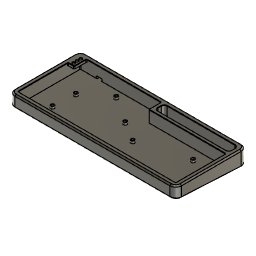
mfrv4n (Autodesk Fusion 360 design; units mm, degrees)
Autodesk Fusion 360 part; units mm, degrees
note: some values were not read from the file. Chosen so that the rebuilt part matches the saved one: a direction. Set by a fixed rule: which sketch regions a step uses.
sketch "PCB Plane Sketch" plane through (0, 0, 0) normal (0, 0, 1) x (1, 0, 0)
  line L0 (0, 0) -> (242.8875, 0) construction
  line L1 (242.8875, 0) -> (242.8875, 76.2) construction
  line L2 (0, 76.2) -> (0, 0) construction
  line L3 (0, 76.2) -> (9.525, 76.2) construction
  line L4 (123.825, 76.2) -> (123.825, 95.25) construction
  line L5 (123.825, 95.25) -> (0, 95.25) construction
  line L6 (0, 95.25) -> (0, 76.2) construction
  line L7 (0, 95.25) -> (9.525, 95.25) construction
  line L8 (9.525, 95.25) -> (9.525, 76.2) construction
  line L9 (9.525, 76.2) -> (0, 76.2) construction
  line L10 (0, 76.2) -> (0, 95.25) construction
  line L11 (242.8875, 76.2) -> (123.825, 76.2) construction
  line L12 (9.525, 76.2) -> (0, 76.2) construction
  line L13 (-0.5, 76.2) -> (-0.5, -0.5)
  line L14 (-0.5, -0.5) -> (243.3875, -0.5)
  line L15 (243.3875, -0.5) -> (243.3875, 76.7)
  line L16 (243.3875, 76.7) -> (124.325, 76.7)
  line L17 (124.325, 76.7) -> (124.325, 95.75)
  line L18 (124.325, 95.75) -> (-0.5, 95.75)
  line L19 (-0.5, 95.75) -> (-0.5, 76.2)
  line L20 (-7.5, 76.2) -> (-7.5, -7.5)
  line L21 (-7.5, -7.5) -> (250.3875, -7.5)
  line L22 (250.3875, -7.5) -> (250.3875, 83.7)
  line L23 (250.3875, 83.7) -> (131.325, 83.7)
  line L24 (131.325, 83.7) -> (131.325, 102.75)
  line L25 (131.325, 102.75) -> (-7.5, 102.75)
  line L26 (-7.5, 102.75) -> (-7.5, 76.2)
  line L27 (131.325, 102.75) -> (250.3875, 102.75)
  line L28 (250.3875, 102.75) -> (250.3875, 83.7)
  dimension "d1" = 242.8875
  dimension "d2" = 76.2
  dimension "d7" = 19.05
  dimension "d8" = 9.525
  dimension "d9" = 123.825
  dimension "d10" = 0.5
  dimension "d11" = 7.5
  constraint horizontal L0
  constraint vertical L1
  constraint vertical L2
  constraint coincident L0.start L2.end
  constraint horizontal L3
  constraint vertical L4
  constraint horizontal L5
  constraint vertical L6
  constraint horizontal L7
  constraint vertical L8
  constraint horizontal L9
  constraint vertical L10
  constraint collinear L11 L12
  constraint perpendicular L22 L27
  constraint perpendicular L23 L28
  measures "d1" distance of L0.start L0.end
  measures "d2" distance of L0.start L2.start
  measures "d7" distance of L2.start L5.end
  measures "d8" distance of L5.end L7.end
  measures "d9" distance of L4 L6
ref_plane "WorkPlane1" through (0, 0, -3.46) normal (0, 0, 1) x (1, 0, 0)
ref_plane "WorkPlane2" through (0, 0, 14.6) normal (0, 0, 1) x (1, 0, 0)
extrude "Extrude1" add sketch "PCB Plane Sketch" along normal blind 14.6 and the other way up to surface (3.46 mm away)
sketch "Base Angle Line Sketch" plane through (250.3875, 0, 0) normal (1, 0, 0) x (0, 1, 0)
  line L0 (102.75, 14.6) -> (-7.5, 14.6)
  line L1 (-7.5, 14.6) -> (-7.5, -3.46)
  line L2 (-7.5, -3.46) -> (102.75, -3.46)
  line L3 (-7.5, 14.6) -> (-7.5, -3.675)
  line L4 (-7.5, -3.675) -> (192.2259, -14.1422)
  line L5 (-7.5, -3.675) -> (192.5, -3.675) construction
  line L6 (102.75, -3.46) -> (102.75, 14.6)
  dimension "d18" = 18.275
  dimension "d19" = 200
  dimension "d20" = 3
  constraint coincident L0.end L1.start
  constraint perpendicular L2 L3
  constraint horizontal L5
  measures "d18" distance of L0.end L3.end
  measures "d19" distance of L3.end L4.end
  measures "d20" angle of L4 L5
ref_plane "WorkPlane3" through (250.3875, 92.363, -8.9086) normal (0, -0.052336, -0.99863) x (0, 0.99863, -0.052336)
sketch "Base Extrude Sketch" plane through (0, 0, -3.46) normal (0, 0, -1) x (1, 0, 0)
  line L0 (124.325, -95.75) -> (-0.5, -95.75)
  line L1 (-0.5, -95.75) -> (-0.5, 0.5)
  line L2 (-0.5, 0.5) -> (243.3875, 0.5)
  line L3 (243.3875, 0.5) -> (243.3875, -76.7)
  line L4 (243.3875, -76.7) -> (124.325, -76.7)
  line L5 (124.325, -76.7) -> (124.325, -95.75)
  line L6 (250.3875, 7.5) -> (-7.5, 7.5)
  line L7 (-7.5, 7.5) -> (-7.5, -102.75)
  line L8 (-7.5, -102.75) -> (250.3875, -102.75)
  line L9 (250.3875, -102.75) -> (250.3875, 7.5)
  line L10 (-0.5, -95.75) -> (124.325, -95.75)
  line L11 (124.325, -76.7) -> (243.3875, -76.7)
  line L12 (243.3875, 0.5) -> (243.3875, -76.7)
  line L13 (243.3875, 0.5) -> (-0.5, 0.5)
  line L14 (-0.5, 0.5) -> (-0.5, -95.75)
  line L15 (124.325, -95.75) -> (124.325, -76.7)
  constraint coincident L0.end L1.start
  constraint coincident L0.start L5.end
  constraint coincident L4.end L5.start
  constraint coincident L3.end L4.start
  constraint coincident L2.end L3.start
  constraint coincident L1.end L2.start
extrude "Extrude2" add sketch "Base Extrude Sketch" along normal up to surface contours L0 L1 L2 L3 L4 L5 L10 L11 L12 L13 L14 L15 | L6 L7 L8 L9 end surface through (250.3875, 92.363, -8.9086) normal (0, -0.052336, -0.99863) offset 0
fillet "Fillet1" radius 9 4 edges at (250.3875, -7.5, 5.4625) (-7.5, -7.5, 5.4625) (250.3875, 102.75, 2.5735) (-7.5, 102.75, 2.5735)
fillet "Fillet2" radius 1 6 edges at (-0.5, 95.75, 5.57) (124.325, 76.7, 5.57) (124.325, 95.75, 5.57) (243.3875, 76.7, 5.57) (243.3875, -0.5, 5.57) (-0.5, -0.5, 5.57)
chamfer "Chamfer1" distance 2 angle 45 8 edges at (121.4438, -7.5, 14.6) (247.7515, -4.864, 14.6) (250.3875, 47.625, 14.6) (247.7515, 100.114, 14.6) (121.4437, 102.75, 14.6) (-4.864, 100.114, 14.6) (-7.5, 47.625, 14.6) (-4.864, -4.864, 14.6)
chamfer "Chamfer2" distance 2 angle 45 8 edges at (250.3875, 47.625, -6.564) (247.7515, 100.114, -9.3148) (121.4437, 102.75, -9.453) (-4.864, 100.114, -9.3148) (-7.5, 47.625, -6.564) (-4.864, -4.864, -3.8131) (121.4438, -7.5, -3.675) (247.7515, -4.864, -3.8131)
extrude "Extrude8" add 1 faces at (161.425, 29.9158, -5.6359) along direction (0, 0.052336, 0.99863) blind 1
sketch "\"Handle\" Cut out Sketch" plane through (0, 0, 14.6) normal (0, 0, 1) x (-1, 0, 0)
  line L0 (-125.325, -76.7) -> (-242.3875, -76.7)
  line L1 (-243.3875, -75.7) -> (-243.3875, -0.5)
  line L2 (-242.3875, 0.5) -> (-0.5, 0.5)
  line L3 (0.5, -0.5) -> (0.5, -94.75)
  line L4 (-0.5, -95.75) -> (-123.325, -95.75)
  line L5 (-124.325, -94.75) -> (-124.325, -77.7)
  line L6 (-1.5, 5.5) -> (-241.3875, 5.5)
  arc A0 (-241.3875, 5.5) -> (-248.3875, -1.5) centre (-241.3875, -1.5) ccw
  line L7 (-248.3875, -1.5) -> (-248.3875, -93.75)
  arc A1 (-248.3875, -93.75) -> (-241.3875, -100.75) centre (-241.3875, -93.75) ccw
  line L8 (-241.3875, -100.75) -> (-1.5, -100.75)
  arc A2 (-1.5, -100.75) -> (5.5, -93.75) centre (-1.5, -93.75) ccw
  line L9 (5.5, -93.75) -> (5.5, -1.5)
  arc A3 (5.5, -1.5) -> (-1.5, 5.5) centre (-1.5, -1.5) ccw
  line L10 (-123.325, -95.75) -> (-243.3875, -95.75) construction
  line L11 (-243.3875, -95.75) -> (-243.3875, -75.7)
  line L12 (-243.3875, -95.75) -> (-129.325, -95.75)
  line L13 (-129.325, -95.75) -> (-129.325, -81.7)
  line L14 (-129.325, -81.7) -> (-243.3875, -81.7)
  line L15 (-243.3875, -81.7) -> (-243.3875, -95.75) construction
  arc A4 (-124.325, -77.7) -> (-125.325, -76.7) centre (-125.325, -77.7) ccw
  arc A5 (-243.3875, -75.7) -> (-242.3875, -76.7) centre (-242.3875, -75.7) ccw
  arc A6 (-242.3875, 0.5) -> (-243.3875, -0.5) centre (-242.3875, -0.5) ccw
  arc A7 (0.5, -0.5) -> (-0.5, 0.5) centre (-0.5, -0.5) ccw
  arc A8 (-0.5, -95.75) -> (0.5, -94.75) centre (-0.5, -94.75) ccw
  arc A9 (-124.325, -94.75) -> (-123.325, -95.75) centre (-123.325, -94.75) ccw
  dimension "d38" = 5
  dimension "d39" = 5
  constraint coincident L4.end L10.start
  constraint coincident L1.start L11.end
  constraint horizontal L12
  constraint vertical L13
  constraint horizontal L14
  constraint vertical L15
  measures "d38" distance of L5 L13
  measures "d39" distance of L0 L14
extrude "Extrude3" cut sketch "\"Handle\" Cut out Sketch" against normal through all contours L11 L12 L13 L14
fillet "Fillet3" radius 4.5 4 edges at (129.325, 95.75, 2.7569) (243.3875, 81.7, 3.1251) (243.3875, 95.75, 2.7569) (129.325, 81.7, 3.1251)
sketch "LED Cover Sketch" plane through (0, 0, 14.6) normal (0, 0, 1) x (-1, 0, 0)
  line L0 (-243.3875, -91.25) -> (-243.3875, -86.2)
  arc A0 (-238.8875, -81.7) -> (-243.3875, -86.2) centre (-238.8875, -86.2) ccw
  line L1 (-238.8875, -81.7) -> (-133.825, -81.7)
  arc A1 (-129.325, -86.2) -> (-133.825, -81.7) centre (-133.825, -86.2) ccw
  line L2 (-129.325, -86.2) -> (-129.325, -91.25)
  arc A2 (-133.825, -95.75) -> (-129.325, -91.25) centre (-133.825, -91.25) ccw
  line L3 (-133.825, -95.75) -> (-238.8875, -95.75)
  arc A3 (-243.3875, -91.25) -> (-238.8875, -95.75) centre (-238.8875, -91.25) ccw
  line L4 (-125.325, -76.7) -> (-242.3875, -76.7)
  line L5 (-243.3875, -75.7) -> (-243.3875, -0.5)
  line L6 (-242.3875, 0.5) -> (-0.5, 0.5)
  line L7 (0.5, -0.5) -> (0.5, -94.75)
  line L8 (-0.5, -95.75) -> (-123.325, -95.75)
  line L9 (-124.325, -94.75) -> (-124.325, -77.7)
  line L10 (-1.5, 5.5) -> (-241.3875, 5.5)
  arc A4 (-241.3875, 5.5) -> (-248.3875, -1.5) centre (-241.3875, -1.5) ccw
  line L11 (-248.3875, -1.5) -> (-248.3875, -93.75)
  arc A5 (-248.3875, -93.75) -> (-241.3875, -100.75) centre (-241.3875, -93.75) ccw
  line L12 (-241.3875, -100.75) -> (-1.5, -100.75)
  arc A6 (-1.5, -100.75) -> (5.5, -93.75) centre (-1.5, -93.75) ccw
  line L13 (5.5, -93.75) -> (5.5, -1.5)
  arc A7 (5.5, -1.5) -> (-1.5, 5.5) centre (-1.5, -1.5) ccw
  arc A8 (-124.325, -77.7) -> (-125.325, -76.7) centre (-125.325, -77.7) ccw
  arc A9 (-243.3875, -75.7) -> (-242.3875, -76.7) centre (-242.3875, -75.7) ccw
  arc A10 (-242.3875, 0.5) -> (-243.3875, -0.5) centre (-242.3875, -0.5) ccw
  arc A11 (0.5, -0.5) -> (-0.5, 0.5) centre (-0.5, -0.5) ccw
  arc A12 (-124.325, -94.75) -> (-123.325, -95.75) centre (-123.325, -94.75) ccw
  line L14 (-28.575, -95.25) -> (-9.525, -95.25) construction
  line L15 (-9.525, -95.25) -> (-9.525, -76.2) construction
  line L16 (-9.525, -76.2) -> (-28.575, -76.2) construction
  line L17 (-28.575, -76.2) -> (-28.575, -95.25) construction
  line L18 (-28.575, -95.25) -> (-9.525, -76.2) construction
  line L19 (-9.525, -95.25) -> (-28.575, -76.2) construction
  line L20 (-9.525, -76.2) -> (0, -76.2) construction
  line L21 (0, -76.2) -> (0, -95.25)
  line L22 (0, -95.25) -> (-9.525, -95.25)
  line L23 (-9.525, -95.25) -> (-9.525, -76.2) construction
  line L24 (-28.575, -85.725) -> (-9.525, -85.725) construction
  circle A13 centre (-4.012, -86.475) radius 1.75
  line L25 (-19.05, -76.2) -> (-19.05, -95.25) construction
  circle A14 centre (-4.012, -92) radius 1.75
  circle A15 centre (-4.012, -80.95) radius 1.75
  line L26 (-26.05, -92.725) -> (-12.05, -92.725) construction
  line L27 (-12.05, -92.725) -> (-12.05, -78.725) construction
  line L28 (-12.05, -78.725) -> (-26.05, -78.725) construction
  line L29 (-26.05, -78.725) -> (-26.05, -92.725) construction
  line L30 (-26.05, -92.725) -> (-12.05, -78.725) construction
  line L31 (-12.05, -92.725) -> (-26.05, -78.725) construction
  line L32 (-9.525, -95.25) -> (-9.525, -95.75) construction
  line L33 (-9.525, -95.75) -> (0.5, -95.75)
  line L34 (0.5, -95.75) -> (0.5, -76.1966)
  line L35 (0.5, -76.1966) -> (0, -76.2) construction
  line L36 (0.5034, -76.6966) -> (0.0017, -76.7)
  line L37 (-9.025, -76.7) -> (0.0017, -76.7)
  line L38 (-9.025, -95.25) -> (-9.025, -76.7)
  line L39 (-9.025, -95.25) -> (-9.025, -95.75)
  point P0 (-19.05, -85.725)
  dimension "d131" = 19.05
  dimension "d132" = 19.05
  dimension "d133" = 9.525
  dimension "d134" = 19.05
  dimension "d135" = 3.5
  dimension "d136" = 0.75
  dimension "d137" = 15.038
  dimension "d139" = 14
  dimension "d140" = 14
  dimension "d141" = 5.525
  dimension "d142" = 5.525
  dimension "d143" = 10.025
  dimension "d148" = -0.5
  constraint horizontal L14
  constraint perpendicular L14 L15
  constraint parallel L14 L16
  constraint parallel L15 L17
  constraint horizontal L20
  constraint vertical L21
  constraint horizontal L22
  constraint vertical L23
  constraint midpoint L17 L24.start
  constraint midpoint L15 L24.end
  constraint midpoint L16 L25.start
  constraint midpoint L14 L25.end
  constraint equal A13 A14
  constraint equal A13 A15
  constraint horizontal L26
  constraint perpendicular L26 L27
  constraint parallel L26 L28
  constraint parallel L27 L29
  constraint coincident L30 P0
  constraint coincident L31 P0
  constraint midpoint L19 P0
  constraint coincident L8 L32.end
  constraint perpendicular L8 L32
  constraint perpendicular L32 L33
  constraint coincident L7 L34.end
  constraint perpendicular L20 L34
  measures "d131" distance of L15.end L16.end
  measures "d132" distance of L14.end L15.end
  measures "d133" distance of L15.end L20.end
  measures "d134" distance of L15.end L14.end
  measures "d135" diameter of A13
  measures "d136" distance of L24 A13.centre
  measures "d137" distance of A13.centre L25
  measures "d139" distance of L27.end L28.end
  measures "d140" distance of L26.end L27.end
  measures "d141" distance of A13.centre A14.centre
  measures "d142" distance of A13.centre A15.centre
  measures "d143" distance of L32.end L33.end
  measures "d148" distance of L35
extrude "Extrude4" add sketch "LED Cover Sketch" against normal blind 4 contours L7 L8 L21 L22 L33 L34 L36 L39 | L21 L22 L37 L38
fillet "Fillet4" radius 1 3 edges at (-0.5, 76.6966, 12.6) (9.025, 76.7, 12.6) (9.025, 95.75, 12.6)
chamfer "Chamfer3" distance 0.5 angle 45 24 edges at (66.675, 95.75, 14.6) (9.3179, 95.4571, 14.6) (9.025, 86.225, 14.6) (8.7321, 76.9929, 14.6) (4.0116, 76.7, 14.6) (-0.3665, 76.3341, 14.6) (-0.5, 38.1675, 14.6) (-0.2071, -0.2071, 14.6) (121.4438, -0.5, 14.6) (243.0946, -0.2071, 14.6) (243.3875, 38.1, 14.6) (243.0946, 76.4071, 14.6) (183.8562, 76.7, 14.6) (124.6179, 76.9929, 14.6) (124.325, 86.225, 14.6) (124.0321, 95.4571, 14.6) (186.3563, 95.75, 14.6) (242.0695, 94.432, 14.6) (243.3875, 88.725, 14.6) (242.0695, 83.018, 14.6) (186.3563, 81.7, 14.6) (130.643, 83.018, 14.6) (129.325, 88.725, 14.6) (130.643, 94.432, 14.6)
chamfer "Chamfer5" distance 0.5 angle 45 3 edges at (5.6436, 80.3172, 14.6) (5.6436, 85.8422, 14.6) (5.6436, 91.3672, 14.6)
sketch "USB C Internal Hole Sketch" plane through (0, 95.75, 0) normal (0, -1, 0) x (1, 0, 0)
  line L0 (123.325, -3.46) -> (123.325, 14.1)
  line L1 (0.5, 10.6) -> (0.5, -3.46)
  line L2 (0.5, -3.46) -> (123.325, -3.46)
  line L3 (0.5, -3.46) -> (0, -3.46) construction
  line L4 (0, -3.46) -> (28.575, -3.46) construction
  line L5 (28.575, -3.46) -> (28.575, 0.2) construction
  line L6 (31.75, 0.2) -> (25.4, 0.2)
  line L7 (23.85, -1.35) -> (23.85, -1.91)
  line L8 (25.4, -3.46) -> (31.75, -3.46)
  line L9 (33.3, -1.91) -> (33.3, -1.35)
  line L10 (33.3, 0.2) -> (23.85, -3.46) construction
  line L11 (23.85, 0.2) -> (33.3, -3.46) construction
  arc A0 (25.4, 0.2) -> (23.85, -1.35) centre (25.4, -1.35) ccw
  arc A1 (33.3, -1.35) -> (31.75, 0.2) centre (31.75, -1.35) ccw
  arc A2 (31.75, -3.46) -> (33.3, -1.91) centre (31.75, -1.91) ccw
  arc A3 (23.85, -1.91) -> (25.4, -3.46) centre (25.4, -1.91) ccw
  line L12 (10.025, 10.6) -> (0.5, 10.6)
  line L13 (123.325, 14.1) -> (10.025, 14.1)
  line L14 (10.025, 14.1) -> (10.025, 10.6)
  point P0 (28.575, -1.63)
  dimension "d70" = 0.5
  dimension "d71" = 28.575
  dimension "d72" = 3.66
  dimension "d73" = 9.45
  dimension "d74" = 3.66
  dimension "d75" = 1.55
  constraint coincident L1.end L2.start
  constraint perpendicular L1 L3
  constraint parallel L2 L4
  constraint perpendicular L4 L5
  constraint horizontal L6
  constraint perpendicular L6 L7
  constraint parallel L6 L8
  constraint parallel L7 L9
  constraint coincident L10 P0
  constraint coincident L11 P0
  constraint midpoint L5 P0
  constraint coincident L11.start L7
  constraint coincident L11.start L6
  constraint tangent L7 A0
  constraint tangent L6 A0
  constraint coincident L10.start L6
  constraint coincident L10.start L9
  constraint tangent L6 A1
  constraint tangent L9 A1
  constraint equal A0 A1
  constraint coincident L11.end L9
  constraint coincident L11.end L8
  constraint tangent L9 A2
  constraint tangent L8 A2
  constraint equal A0 A2
  constraint coincident L10.end L8
  constraint coincident L10.end L7
  constraint tangent L8 A3
  constraint tangent L7 A3
  constraint equal A0 A3
  measures "d70" distance of L1.end L3.end
  measures "d71" distance of L3.end L4.end
  measures "d72" distance of L4.end L5.end
  measures "d73" distance of L10.end L11.end
  measures "d74" distance of L11.start L10.end
  measures "d75" radius of A0
extrude "Extrude5" cut sketch "USB C Internal Hole Sketch" against normal blind 8.5 contours L2 L6 L7 L8 L9 A0 A1 A2 A3
sketch "USB C External Hole Sketch" plane through (0, 102.75, 0) normal (0, 1, 0) x (-1, 0, 0)
  line L0 (-25.4, -3.46) -> (-31.75, -3.46)
  arc A0 (-33.3, -1.91) -> (-31.75, -3.46) centre (-31.75, -1.91) ccw
  line L1 (-33.3, -1.91) -> (-33.3, -1.35)
  arc A1 (-31.75, 0.2) -> (-33.3, -1.35) centre (-31.75, -1.35) ccw
  line L2 (-31.75, 0.2) -> (-25.4, 0.2)
  arc A2 (-23.85, -1.35) -> (-25.4, 0.2) centre (-25.4, -1.35) ccw
  line L3 (-23.85, -1.35) -> (-23.85, -1.91)
  arc A3 (-25.4, -3.46) -> (-23.85, -1.91) centre (-25.4, -1.91) ccw
  line L4 (-241.3875, -7.453) -> (-1.5, -7.453)
  line L5 (-1.5, -7.453) -> (-1.5, 12.6)
  line L6 (-1.5, 12.6) -> (-241.3875, 12.6)
  line L7 (-241.3875, 12.6) -> (-241.3875, -7.453)
  line L8 (-28.575, 0.2) -> (-28.575, -3.46) construction
  line L9 (-25.4, 2.45) -> (-31.75, 2.45)
  line L10 (-35.55, -1.35) -> (-35.55, -1.91)
  line L11 (-31.75, -5.71) -> (-25.4, -5.71)
  line L12 (-21.6, -1.91) -> (-21.6, -1.35)
  line L13 (-21.6, 2.45) -> (-35.55, -5.71) construction
  line L14 (-35.55, 2.45) -> (-21.6, -5.71) construction
  arc A4 (-31.75, 2.45) -> (-35.55, -1.35) centre (-31.75, -1.35) ccw
  arc A5 (-21.6, -1.35) -> (-25.4, 2.45) centre (-25.4, -1.35) ccw
  arc A6 (-25.4, -5.71) -> (-21.6, -1.91) centre (-25.4, -1.91) ccw
  arc A7 (-35.55, -1.91) -> (-31.75, -5.71) centre (-31.75, -1.91) ccw
  point P0 (-28.575, -1.63)
  dimension "d78" = 13.95
  dimension "d79" = 8.16
  dimension "d80" = 3.8
  constraint midpoint L2 L8.start
  constraint midpoint L0 L8.end
  constraint horizontal L9
  constraint perpendicular L9 L10
  constraint parallel L9 L11
  constraint parallel L10 L12
  constraint coincident L13 P0
  constraint coincident L14 P0
  constraint midpoint L8 P0
  constraint coincident L14.start L10
  constraint coincident L14.start L9
  constraint tangent L10 A4
  constraint tangent L9 A4
  constraint coincident L13.start L9
  constraint coincident L13.start L12
  constraint tangent L9 A5
  constraint tangent L12 A5
  constraint equal A4 A5
  constraint coincident L14.end L12
  constraint coincident L14.end L11
  constraint tangent L12 A6
  constraint tangent L11 A6
  constraint equal A4 A6
  constraint coincident L13.end L11
  constraint coincident L13.end L10
  constraint tangent L11 A7
  constraint tangent L10 A7
  constraint equal A4 A7
  measures "d78" distance of L13.end L14.end
  measures "d79" distance of L14.start L13.end
  measures "d80" radius of A4
extrude "Extrude6" cut sketch "USB C External Hole Sketch" against normal blind 3.5 contours L9 L10 L11 L12 A4 A5 A6 A7
chamfer "Chamfer6" distance 0.25 angle 45 8 edges at (34.437, 102.75, 1.337) (28.575, 102.75, 2.45) (22.713, 102.75, 1.337) (21.6, 102.75, -1.63) (22.713, 102.75, -4.597) (28.575, 102.75, -5.71) (34.437, 102.75, -4.597) (35.55, 102.75, -1.63)
sketch "Screw Holes Sketch" plane through (0, 0, 0) normal (0, 0, 1) x (1, 0, 0)
  circle A0 centre (66.675, 84.1375) radius 2.75
  line L0 (0, 95.25) -> (0, 76.2)
  line L1 (123.825, 95.25) -> (0, 95.25)
  line L2 (0, 76.2) -> (19.05, 76.2) construction
  line L3 (19.05, 76.2) -> (19.05, 95.25) construction
  line L4 (19.05, 95.25) -> (0, 95.25) construction
  line L5 (0, 95.25) -> (0, 76.2) construction
  line L6 (0, 76.2) -> (19.05, 76.2) construction
  line L7 (19.05, 76.2) -> (19.05, 57.15) construction
  line L8 (19.05, 57.15) -> (0, 57.15) construction
  line L9 (0, 57.15) -> (0, 76.2) construction
  line L10 (0, 76.2) -> (19.05, 57.15) construction
  line L11 (0, 57.15) -> (19.05, 76.2) construction
  circle A1 centre (31.325, 57.15) radius 2.75
  circle A2 centre (107.525, 57.15) radius 2.75
  circle A3 centre (210.575, 59.276) radius 2.75
  circle A4 centre (182.325, 10.641) radius 2.75
  circle A5 centre (76.675, 10.926) radius 2.75
  circle A6 centre (29.725, 22.376) radius 2.75
  line L12 (0, 66.675) -> (19.05, 66.675) construction
  line L13 (9.525, 76.2) -> (9.525, 57.15) construction
  circle A7 centre (138.175, 38.1) radius 2.75
  dimension "d84" = 5.5
  dimension "d85" = 66.675
  dimension "d86" = 11.1125
  dimension "d87" = 19.05
  dimension "d88" = 19.05
  dimension "d89" = 19.05
  dimension "d90" = 9.525
  dimension "d91" = 21.8
  dimension "d92" = 20.2
  dimension "d93" = 44.299
  dimension "d94" = 9.525
  dimension "d95" = 98
  dimension "d96" = 67.15
  dimension "d97" = 55.749
  dimension "d98" = 7.399
  dimension "d99" = 201.05
  dimension "d100" = 172.8
  dimension "d101" = 56.034
  dimension "d102" = 128.65
  dimension "d103" = 28.575
  constraint horizontal L2
  constraint vertical L3
  constraint horizontal L4
  constraint vertical L5
  constraint coincident L0.end L2.start
  constraint horizontal L6
  constraint vertical L7
  constraint horizontal L8
  constraint vertical L9
  constraint perpendicular L10 L11
  constraint equal A0 A1
  constraint equal A0 A6
  constraint equal A0 A2
  constraint equal A0 A5
  constraint equal A0 A3
  constraint equal A0 A4
  constraint midpoint L9 L12.start
  constraint midpoint L7 L12.end
  constraint midpoint L6 L13.start
  constraint midpoint L8 L13.end
  constraint equal A0 A7
  measures "d84" diameter of A0
  measures "d85" distance of A0.centre L0
  measures "d86" distance of A0.centre L1
  measures "d87" distance of L0.end L2.end
  measures "d88" distance of L0.end L0.start
  measures "d89" distance of L0.end L8.end
  measures "d90" distance of A1.centre L12
  measures "d91" distance of A1.centre L13
  measures "d92" distance of A6.centre L13
  measures "d93" distance of A6.centre L12
  measures "d94" distance of A2.centre L12
  measures "d95" distance of A2.centre L13
  measures "d96" distance of A5.centre L13
  measures "d97" distance of A5.centre L12
  measures "d98" distance of A3.centre L12
  measures "d99" distance of A3.centre L13
  measures "d100" distance of A4.centre L13
  measures "d101" distance of A4.centre L12
  measures "d102" distance of L13 A7.centre
  measures "d103" distance of L12 A7.centre
extrude "Extrude7" add sketch "Screw Holes Sketch" against normal up to surface (3.46 mm away)
hole "Hole1" at (31.325, 57.15, 0) direction (0, 0, -1) diameter 3.2 depth 4 tip angle 180
hole "Hole2" at (66.675, 84.1375, 0) direction (0, 0, -1) diameter 3.2 depth 4 tip angle 180
hole "Hole3" at (107.525, 57.15, 0) direction (0, 0, -1) diameter 3.2 depth 4 tip angle 180
hole "Hole4" at (29.725, 22.376, 0) direction (0, 0, -1) diameter 3.2 depth 4 tip angle 180
hole "Hole5" at (76.675, 10.926, 0) direction (0, 0, -1) diameter 3.2 depth 4 tip angle 180
hole "Hole6" at (138.175, 38.1, 0) direction (0, 0, -1) diameter 3.2 depth 4 tip angle 180
hole "Hole7" at (182.325, 10.641, 0) direction (0, 0, -1) diameter 3.2 depth 4 tip angle 180
hole "Hole8" at (210.575, 59.276, 0) direction (0, 0, -1) diameter 3.2 depth 4 tip angle 180
move_body "Move1" [suppressed]
equation "d1 = ( 19.05 * 12.75 ) * 1 mm"
equation "d2 = ( 19.05 * 4 ) * 1 mm"
equation "d8 = 19.05 mm * 0.5"
equation "d9 = 19.05 mm * 6.5"
equation "d71 = 19.05 mm * 1.5"
equation "d73 = ( 4.725 * 2 ) * 1 mm"
equation "d85 = 3.5 * 19.05 mm"
equation "d86 = ( 19.05 / 2 ) * 1 mm + 1.5875 mm"
equation "d133 = 19.05 mm * 0.5"
equation "d143 = 19.05 mm * 0.5 + 0.5 mm"
